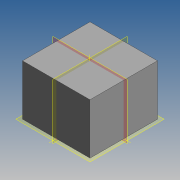
# Autodesk Inventor part: P022_Coque_boitier
Saved by Autodesk Inventor 2021.3 (Build 253353000, 353)
## iProperties
Created: 2021-11-18
Part Number: P022_Coque_boitier
Material: Générique
Document SubType Name: Modeling
Designer: gabri
Density: 1 g/cm^3
Appearance: Par défaut
Author: gabri
Autodesk Inventor part; units mm, degrees
sketch "Sketch2" plane through (0, 0, 0) normal (0, 0, 1) x (1, 0, 0)
  line L0 (100, -100) -> (-100, -100)
  line L1 (-100, -100) -> (-100, 100)
  line L2 (-100, 100) -> (100, 100)
  line L3 (100, 100) -> (100, -100)
  line L4 (100, -100) -> (-100, 100) construction
  line L5 (-100, -100) -> (100, 100) construction
  point P0 (0, 0)
  dimension "d0" = 200
  dimension "d1" = 200
  constraints: 12 end point, 2 midpoint, 2 parallel, 1 horizontal, 1 perpendicular
  measures "d0" distance of L1.end L2.end
  measures "d1" distance between parallel lines of L0 L2
extrude "Extrusion1" add sketch "Sketch2" along normal blind 150
sketch "Sketch3" plane through (0, 0, 0) normal (0, 0, -1) x (-1, 0, 0)
  line L0 (-97, 97) -> (97, 97)
  line L1 (97, 97) -> (97, -97)
  line L2 (97, -97) -> (-97, -97)
  line L3 (-97, -97) -> (-97, 97)
  line L4 (-97, 97) -> (97, -97) construction
  line L5 (97, 97) -> (-97, -97) construction
  line L6 (-100, 100) -> (100, 100) construction
  line L7 (-100, -100) -> (-100, 100) construction
  line L8 (100, -100) -> (-100, -100) construction
  line L9 (100, 100) -> (100, -100) construction
  point P0 (0, 0)
  dimension "d4" = 3
  dimension "d5" = 3
  constraints: 12 end point, 2 midpoint, 2 parallel, 1 horizontal, 1 perpendicular
  measures "d4" distance between parallel lines of L8 L2
  measures "d5" distance between parallel lines of L7 L3
extrude "Extrusion2" cut sketch "Sketch3" against normal blind 147
sketch "Sketch4" plane through (-100, -100, 0) normal (-1, 0, 0) x (0, 0, 1)
  line L0 (0, 200) -> (0, 0) construction
  line L1 (0, 0) -> (150, 0) construction
  line L2 (150, 200) -> (150, 0) construction
  line L3 (0, 200) -> (150, 200) construction
  line L4 (38.5, 116) -> (81.5, 116)
  line L5 (81.5, 116) -> (81.5, 184)
  line L6 (81.5, 184) -> (38.5, 184)
  line L7 (38.5, 184) -> (38.5, 116)
  line L8 (38.5, 116) -> (81.5, 184) construction
  line L9 (81.5, 116) -> (38.5, 184) construction
  circle A0 centre (60, 50) radius 25
  line L10 (0, 200) -> (0, 0) construction
  point P0 (0, 100)
  point P1 (60, 150)
  dimension "d8" = 43
  dimension "d9" = 68
  dimension "d10" = 50
  dimension "d11" = 60
  dimension "d12" = 60
  dimension "d13" = 200
  dimension "d14" = 50
  dimension "d15" = 50
  constraints: 12 end point, 2 midpoint, 2 parallel, 1 centre point, 1 horizontal, 1 perpendicular
  measures "d8" distance between parallel lines of L7 L5
  measures "d9" distance between parallel lines of L4 L6
  measures "d10" diameter of A0
  measures "d11" distance from line of L0 A0.centre
  measures "d12" distance from line of L0 point (60, 150)
  measures "d13" distance between parallel lines of L1 L3
  measures "d14" distance from line of L3 point (60, 150)
  measures "d15" distance from line of L1 A0.centre
extrude "Extrusion3" cut sketch "Sketch4" against normal up to surface (3 mm away)
sketch "Sketch5" plane through (-100, -100, 0) normal (0, -1, 0) x (1, 0, 0)
  point P0 (100, 0)
equation "\"d14\" = 0.25 * d13"
equation "\"d15\" = 0.25 * d13"
body "Solid1"
